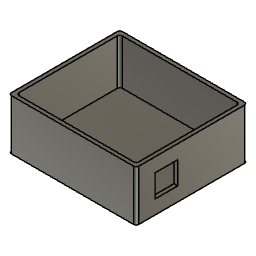
Edl_box_ (Autodesk Fusion 360 design; units mm, degrees)
Autodesk Fusion 360 part; units mm, degrees
sketch "Sketch1" plane through (0, 0, 0) normal (0, 0, 1) x (1, 0, 0)
  line L0 (-35, 30) -> (60, 30)
  line L1 (60, 30) -> (60, -52)
  line L2 (60, -52) -> (-35, -52)
  line L3 (-35, -52) -> (-35, 30)
  line L4 (-38, 33) -> (63, 33)
  line L5 (63, 33) -> (63, -55)
  line L6 (63, -55) -> (-38, -55)
  line L7 (-38, -55) -> (-38, 33)
  dimension "d1" = 82
  dimension "d2" = 95
  dimension "d3" = 3
  dimension "d4" = 3
  dimension "d5" = 3
  dimension "d6" = 3
  constraint horizontal L0
  constraint perpendicular L0 L1
  constraint perpendicular L1 L2
  constraint perpendicular L0 L3
  constraint horizontal L4
  constraint perpendicular L4 L5
  constraint perpendicular L5 L6
  constraint perpendicular L4 L7
  measures "d1" distance of L0 L2
  measures "d2" distance of L1 L3
  measures "d3" distance of L0 L4
  measures "d4" distance of L3 L7
  measures "d5" distance of L2 L6
  measures "d6" distance of L1 L5
extrude "Extrude1" add sketch "Sketch1" along normal blind 40
extrude "Extrude2" add sketch "Sketch1" along normal blind 4 contours L0 L1 L2 L3
sketch "Sketch2" plane through (63, 0, 0) normal (1, 0, 0) x (0, 1, 0)
  line L0 (-55, 0) -> (33, 0)
  line L1 (33, 0) -> (33, 40)
  line L2 (33, 40) -> (-55, 40)
  line L3 (-55, 40) -> (-55, 0)
  line L4 (-22, 29) -> (-40, 29)
  line L5 (-40, 29) -> (-40, 11)
  line L6 (-40, 11) -> (-22, 11)
  line L7 (-22, 11) -> (-22, 29)
  line L8 (-22, 29) -> (-40, 11) construction
  line L9 (-40, 29) -> (-22, 11) construction
  point P0 (-31, 20)
  dimension "d11" = 18
  dimension "d12" = 18
  dimension "d13" = 15
  dimension "d14" = 11
  constraint horizontal L4
  constraint perpendicular L4 L5
  constraint parallel L4 L6
  constraint parallel L5 L7
  constraint coincident L8 P0
  constraint coincident L9 P0
  measures "d11" distance of L5.end L6.end
  measures "d12" distance of L4.end L5.end
  measures "d13" distance of L3 L5
  measures "d14" distance of L0 L6
extrude "Extrude3" cut sketch "Sketch2" against normal blind 3 contours L4 L5 L6 L7
fillet "Fillet1" radius 2 1 edges at (63, -55, 20)
fillet "Fillet2" radius 2 1 edges at (63, 33, 20)
fillet "Fillet3" radius 2 1 edges at (-38, 33, 20)
fillet "Fillet4" radius 2 1 edges at (-38, -55, 20)
fillet "Fillet5" radius 2 1 edges at (-35, 30, 22)
fillet "Fillet6" radius 2 1 edges at (-35, -52, 22)
fillet "Fillet7" radius 2 1 edges at (60, -52, 22)
fillet "Fillet8" radius 2 1 edges at (60, 30, 22)
